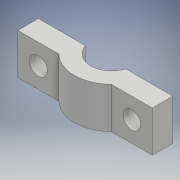
# Autodesk Inventor part: clampCap
Saved by Autodesk Inventor 2018 (Build 220112000, 112)
## iProperties
Created: 2018-11-24
Part Number: clampCap
Material: Generic
Document SubType Name: Modeling
Designer: Prakash
Density: 1 g/cm^3
Appearance: Default
Author: Prakash
Autodesk Inventor part; units mm, degrees
ref_plane "YZ Plane" through (0, 0, 0) normal (1, 0, 0) x (0, 1, 0)
ref_plane "XZ Plane" through (0, 0, 0) normal (0, 1, 0) x (-1, 0, 0)
ref_plane "XY Plane" through (0, 0, 0) normal (0, 0, 1) x (1, 0, 0)
sketch "Sketch1" plane through (0, 0, 0) normal (0, 0, 1) x (1, 0, 0)
  line L0 (0, 0) -> (10, 0)
  line L1 (0, 0) -> (0, 5)
  line L2 (0, 5) -> (11.504, 5)
  arc A0 (11.504, 5) -> (21.3051, 5) centre (16.4046, 6.5) ccw
  arc A1 (10, 0) -> (22.8091, 0) centre (16.4046, 6.5) ccw
  line L3 (21.3051, 5) -> (32.8091, 5)
  line L4 (32.8091, 5) -> (32.8091, 0)
  line L5 (32.8091, 0) -> (22.8091, 0)
  dimension "d0" = 10
  dimension "d1" = 11.504
  dimension "d2" = 5
  dimension "d3" = 5.125
  dimension "d4" = 1.5
  constraints: 12 end point, 4 point on circle, 3 collinear, 2 centre point, 2 horizontal, 2 perpendicular, 1 coincident, 1 vertical
  measures "d0" distance of L0.start L0.end
  measures "d1" distance of L1.end L2.end
  measures "d2" distance between parallel lines of L0 L2
  measures "d3" radius of A0
  measures "d4" distance from line of L2 A0.centre
extrude "Extrusion1" add sketch "Sketch1" along normal blind 10
sketch "Sketch2" plane through (22.8091, 0, 0) normal (0, -1, 0) x (1, 0, 0)
  line L0 (0, 0) -> (10, 0) projected
  line L1 (10, 0) -> (10, 10) projected
  line L2 (0, 10) -> (10, 10) projected
  line L3 (0, 0) -> (0, 10) projected
  line L4 (-22.8091, 0) -> (-12.8091, 0) projected
  line L5 (-12.8091, 0) -> (-12.8091, 10) projected
  line L6 (-22.8091, 10) -> (-12.8091, 10) projected
  line L7 (-22.8091, 0) -> (-22.8091, 10) projected
  line L8 (-22.8091, 0) -> (-22.8091, 10) projected
  line L9 (-22.8091, 10) -> (-12.8091, 0)
  line L10 (-22.8091, 0) -> (-12.8091, 10)
  line L11 (0, 10) -> (10, 0)
  line L12 (0, 0) -> (10, 0) projected
  line L13 (0, 0) -> (10, 10)
  point P0 (-17.8091, 5)
  point P1 (5, 5)
  constraints: 8 end point, 3 perpendicular, 2 midpoint, 2 point on line
hole "Hole1" at (5, 0, 5) at (27.8091, 0, 5) direction (0, 1, 0) diameter 4.305 end through all clearance for "Flat Head Machine Screw (82)" size "#6" standard "Ansi Unified Screw Threads"
body "Solid1"
